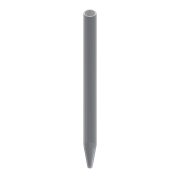
# Autodesk Inventor part: Pipette
Saved by Autodesk Inventor 2015 SP2 (Build 190223200, 223)
## iProperties
Created: 2016-12-12
Part Number: Pipette
Material: Glass
Document SubType Name: Modeling
Designer: dsnyder
Density: 2.18 g/cm^3
Appearance: Clear
Author: dsnyder
Autodesk Inventor part; units mm, degrees
ref_plane "YZ Plane" through (0, 0, 0) normal (1, 0, 0) x (0, 1, 0)
ref_plane "XZ Plane" through (0, 0, 0) normal (0, 1, 0) x (-1, 0, 0)
ref_plane "XY Plane" through (0, 0, 0) normal (0, 0, 1) x (1, 0, 0)
sketch "Sketch1" plane through (0, 0, 0) normal (0, 0, 1) x (1, 0, 0)
  line L0 (0, 0) -> (1.27, 0)
  line L1 (3.175, 12.7) -> (3.175, 90.4875)
  line L2 (3.175, 90.4875) -> (0, 90.4875)
  line L3 (0, 90.4875) -> (0, 0)
  line L4 (1.27, 0) -> (3.175, 12.7)
  dimension "d0" = 3.175
  dimension "d1" = 77.7875
  dimension "d2" = 1.27
  dimension "d3" = 12.7
  constraints: 10 end point, 2 parallel, 1 horizontal, 1 perpendicular
  measures "d0" distance of L2.end L1.end
  measures "d1" distance of L1.end L1.start
  measures "d2" distance of L0.end L0.start
  measures "d3" distance from line of L1.start L0
revolve "Revolution1" add sketch "Sketch1" angle 360 about axis through (0, 90.4875, 0) along (0, -1, 0)
shell "Shell1" thickness 0.635 removed faces 2 at (-0.5202, 90.4875, -0.7796) at (-0.1274, 0, 0.3526)
fillet "Fillet1" radius 3.175 1 edges at (-3.175, 12.7, 0)
body "Solid1"
